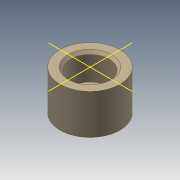
# Autodesk Inventor part: Standard
Saved by Autodesk Inventor 2020.3 (Build 243373000, 373)
## iProperties
RuleStatus: InUse
AfterDocSave0: file://Part Number Cleaner
Created: 2023-02-27
Material: ABS, BEIGE
Catalog Web Link: https://www.janelia.org/
Vendor: HHMI: JRC - jET
Document SubType Name: Modeling
Designer: arnoldj
Density: 1.06 g/cm^3
Appearance: Beige
DESIGN DEPARTMENT: HHMI: JRC - jET
ALTERED ITEM PART NUMBER: N/A
ALTERED ITEM VENDOR: N/A
ALTERED ITEM DESCRIPTION: N/A
Title: Standard
Author: arnoldj
Revision Number: 0
Autodesk Inventor part; units mm, degrees
ref_plane "YZ Plane" through (0, 0, 0) normal (1, 0, 0) x (0, 1, 0)
ref_plane "XZ Plane" through (0, 0, 0) normal (0, 1, 0) x (-1, 0, 0)
ref_plane "XY Plane" through (0, 0, 0) normal (0, 0, 1) x (1, 0, 0)
sketch "Sketch1" plane through (0, 0, 0) normal (0, 1, 0) x (-1, 0, 0)
  line L0 (0, -20.0025) -> (0, 20.0025) projected
  line L1 (-20.0025, 0) -> (20.0025, 0) projected
  circle A0 centre (0, 0) radius 14.2875
  dimension "d0" = 28.575
  constraints: 1 centre point, 1 coincident
  measures "d0" diameter of A0
extrude "Extrusion1" add sketch "Sketch1" along normal blind 19.05
sketch "Sketch2" plane through (0, 19.05, 0) normal (0, 1, 0) x (1, 0, 0)
  line L0 (0, 20.0025) -> (0, -20.0025) projected
  line L1 (20.0025, 0) -> (-20.0025, 0) projected
  point P0 (0, 0)
sketch "Sketch3" plane through (0, 19.05, 0) normal (0, 1, 0) x (1, 0, 0)
  point P0 (0, 0)
hole "Hole1" at (0, 19.05, 0) direction (0, -1, 0) diameter 6.35 end through all counterbore diameter 18.288 counterbore depth 12.7
chamfer "Chamfer1" distance 1.27 angle 45 1 edges at (0, 19.05, -9.144)
body "Solid1"
